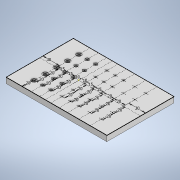
# Autodesk Inventor part: Testpad
Saved by Autodesk Inventor 2020.3 (Build 243373000, 373)
## iProperties
Created: 2021-04-12
Part Number: Testpad
Material: Generic
Document SubType Name: Modeling
Designer: sanyi
Density: 1 g/cm^3
Appearance: Default
Author: sanyi
Autodesk Inventor part; units mm, degrees
ref_plane "YZ Plane" through (0, 0, 0) normal (1, 0, 0) x (0, 1, 0)
ref_plane "XZ Plane" through (0, 0, 0) normal (0, 1, 0) x (-1, 0, 0)
ref_plane "XY Plane" through (0, 0, 0) normal (0, 0, 1) x (1, 0, 0)
sketch "Sketch1" plane through (0, 0, 0) normal (0, 1, 0) x (-1, 0, 0)
  line L0 (70, 60) -> (-110, 60)
  line L1 (-110, 60) -> (-110, -60)
  line L2 (-110, -60) -> (70, -60)
  line L3 (70, -60) -> (70, 60)
  line L4 (0, 60) -> (0, -60) construction
  line L5 (70, 0) -> (-110, 0) construction
  line L6 (40, 60) -> (40, -60) construction
  line L7 (25, 60) -> (25, -60) construction
  line L8 (10, 60) -> (10, -60) construction
  line L9 (-10, 60) -> (-10, -60) construction
  line L10 (-25, 60) -> (-25, -60) construction
  line L11 (-40, 60) -> (-40, -60) construction
  line L12 (-60, 60) -> (-60, -60) construction
  line L13 (-80, 60) -> (-80, -60) construction
  point P0 (0, 0)
  point P1 (40, 0)
  point P2 (25, 0)
  point P3 (10, 0)
  point P4 (-10, 0)
  point P5 (-25, 0)
  point P6 (-40, 0)
  point P7 (-60, 0)
  point P8 (-80, 0)
  point P9 (40, 20)
  point P10 (40, 40)
  point P11 (25, 20)
  point P12 (25, 40)
  point P13 (10, 20)
  point P14 (10, 40)
  point P15 (-25, 40)
  point P16 (-25, 20)
  point P17 (-40, 40)
  point P18 (-40, 20)
  point P19 (-60, 40)
  point P20 (-60, 20)
  point P21 (-80, 40)
  point P22 (-80, 20)
  point P23 (-10, 40)
  point P24 (-10, 20)
  point P25 (40, -20)
  point P26 (40, -40)
  point P27 (25, -20)
  point P28 (25, -40)
  point P29 (10, -20)
  point P30 (10, -40)
  point P31 (-25, -40)
  point P32 (-25, -20)
  point P33 (-40, -40)
  point P34 (-40, -20)
  point P35 (-60, -40)
  point P36 (-60, -20)
  point P37 (-80, -40)
  point P38 (-80, -20)
  point P39 (-10, -40)
  point P40 (-10, -20)
  dimension "d6" = 10
  dimension "d8" = 15
  dimension "d9" = 15
  dimension "d10" = 30
  dimension "d11" = 10
  dimension "d12" = 15
  dimension "d13" = 15
  dimension "d14" = 20
  dimension "d15" = 20
  dimension "d16" = 30
  dimension "d17" = 20
  dimension "d18" = 20
  dimension "d19" = 20
  dimension "d22" = 20
  dimension "d23" = 20
  dimension "d24" = 20
  dimension "d25" = 20
  dimension "d29" = 20
  dimension "d30" = 20
  dimension "d31" = 20
  dimension "d32" = 20
  dimension "d33" = 20
  dimension "d34" = 20
  dimension "d35" = 20
  dimension "d36" = 20
  dimension "d37" = 20
  dimension "d38" = 20
  constraints: 22 end point, 16 point on line, 16 vertical alignment, 11 midpoint, 9 parallel, 2 vertical, 36 other
  measures "d6" distance from line of L4 point (10, 0)
  measures "d8" distance of point (25, 0) point (40, 0)
  measures "d9" distance of point (10, 0) point (25, 0)
  measures "d10" distance from line of L3 point (40, 0)
  measures "d11" distance from line of L4 point (-10, 0)
  measures "d12" distance of point (-25, 0) point (-10, 0)
  measures "d13" distance of point (-40, 0) point (-25, 0)
  measures "d14" distance of point (-60, 0) point (-40, 0)
  measures "d15" distance of point (-80, 0) point (-60, 0)
  measures "d16" distance from line of L1 point (-80, 0)
  measures "d17" distance of point (40, 0) point (40, 20)
  measures "d18" distance of point (40, 40) point (40, 20)
  measures "d22" distance of point (25, 0) point (25, 20)
  measures "d23" distance of point (25, 40) point (25, 20)
  measures "d24" distance of point (10, 20) point (10, 40)
  measures "d25" distance of point (10, 0) point (10, 20)
  measures "d29" distance of point (-25, 20) point (-25, 40)
  measures "d30" distance of point (-25, 0) point (-25, 20)
  measures "d31" distance of point (-40, 20) point (-40, 40)
  measures "d32" distance of point (-40, 0) point (-40, 20)
  measures "d33" distance of point (-60, 20) point (-60, 40)
  measures "d34" distance of point (-60, 0) point (-60, 20)
  measures "d35" distance of point (-80, 40) point (-80, 20)
  measures "d36" distance of point (-80, 0) point (-80, 20)
  measures "d37" distance of point (-10, 20) point (-10, 0)
  measures "d38" distance of point (-10, 40) point (-10, 20)
extrude "Extrusion1" add sketch "Sketch1" against normal blind 10
hole "Hole1" at (-40, 0, 40) direction (0, -1, 0) diameter 5.6 depth 6.5 counterbore diameter 9 counterbore depth 1
hole "Hole2" at (-25, 0, 40) at (-10, 0, 40) direction (0, -1, 0) diameter 5.6 depth 6.5
hole "Hole3" at (-40, 0, 20) direction (0, -1, 0) diameter 5.8 depth 6.5 counterbore diameter 9 counterbore depth 1
hole "Hole4" at (-25, 0, 20) at (-10, 0, 20) direction (0, -1, 0) diameter 5.8 depth 6.5
hole "Hole5" at (-40, 0, 0) direction (0, -1, 0) diameter 5.9 depth 6.5 counterbore diameter 9 counterbore depth 1
hole "Hole6" at (-25, 0, 0) at (-10, 0, 0) direction (0, -1, 0) diameter 5.9 depth 6.5
hole "Hole7" at (-40, 0, -20) direction (0, -1, 0) diameter 6 depth 6.5 counterbore diameter 9 counterbore depth 1
hole "Hole8" at (-25, 0, -20) at (-10, 0, -20) direction (0, -1, 0) diameter 6 depth 6.5
hole "Hole9" at (-40, 0, -40) direction (0, -1, 0) diameter 6.2 depth 6.5 counterbore diameter 9 counterbore depth 1
hole "Hole10" at (-25, 0, -40) at (-10, 0, -40) direction (0, -1, 0) diameter 6.2 depth 6.5
hole "Hole11" at (80, 0, -40) direction (0, -1, 0) diameter 2.2 end through all
hole "Hole12" at (80, 0, -20) direction (0, -1, 0) diameter 2 end through all
hole "Hole13" at (80, 0, 0) direction (0, -1, 0) diameter 1.9 end through all
hole "Hole14" at (80, 0, 20) direction (0, -1, 0) diameter 1.8 end through all
hole "Hole15" at (80, 0, 40) direction (0, -1, 0) diameter 1.6 end through all
hole "Hole16" at (60, 0, 40) direction (0, -1, 0) diameter 1.6 end through all
hole "Hole17" at (60, 0, 20) direction (0, -1, 0) diameter 1.7 end through all
hole "Hole18" at (60, 0, 0) direction (0, -1, 0) diameter 1.8 end through all
hole "Hole19" at (60, 0, -20) direction (0, -1, 0) diameter 1.9 end through all
hole "Hole20" at (60, 0, -40) direction (0, -1, 0) diameter 2 end through all
hole "Hole21" at (10, 0, 20) at (25, 0, 20) at (40, 0, 20) direction (0, -1, 0) diameter 3 depth 3.2
hole "Hole22" at (10, 0, 0) at (25, 0, 0) at (40, 0, 0) direction (0, -1, 0) diameter 3.1 depth 3.2
hole "Hole23" at (10, 0, -20) at (25, 0, -20) at (40, 0, -20) direction (0, -1, 0) diameter 3.2 depth 3.2
hole "Hole24" at (10, 0, -40) at (25, 0, -40) at (40, 0, -40) direction (0, -1, 0) diameter 3.3 depth 3.2
hole "Hole25" at (25, 0, 40) at (40, 0, 40) at (10, 0, 40) direction (0, -1, 0) diameter 2.9 depth 3.2
body "Solid1"
